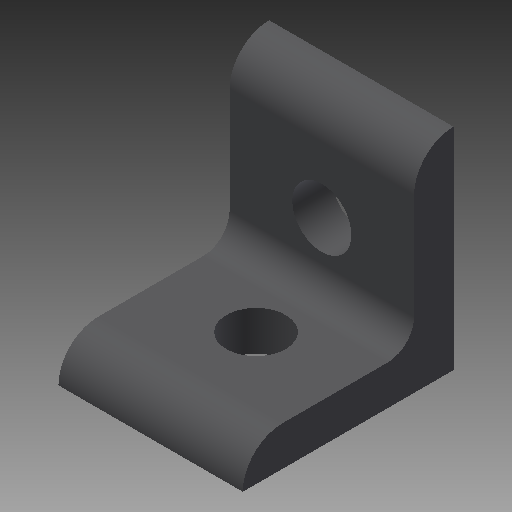
# Autodesk Inventor part: 4119
Saved by Autodesk Inventor 2017 SP1 (Build 210196100, 196)
## iProperties
Category: PARTsolutions
Company: 8020
Created: 2016-04-09
Part Number: 4119
Catalog Web Link: www.cadenas.de
Description: 4119, 4302-Joining Plates - 2 Hole Inside Corner Bracket
Vendor: 8020
Document SubType Name: Modeling
Designer: psAdmin
Manufacturer: 8020
Mass: 4.32354 g
Surface Area: 26.1381 cm^2
Volume: 4.32354 cm^3
Density: 1 g/cm^3
Material: Generic
Appearance: PSOLRGB-175-175-175
PSOL_IDENT_0: {$CADENAS_DATA\23d-libs\8020\inch\joining_plates\4119.prj},154 {VTYP=3D},{NB=4119},{LINA=4119},{NN=4
PSOL_IDENT_1: 119, 4302},{DATE=26.07.2013 08:18:18},{GEOMDATE=02.12.2011 13:06:00},{VERSION=},{LINEID=10},{LINESUB
PSOL_IDENT_2: ID=-1},{WBVAR=}  {NB=4119},{LINA=4119},{KT=DUMMY},{PN=4119},{A=0.875},{B=1.000},{C=1.000},{D=0.188},
PSOL_IDENT_3: {D1=0.18750},{E=0.281},{W=.025},{R=0.125}
NN: 4119, 4302
NT: Joining Plates - 2 Hole Inside Corner Bracket
NB: 4119
NBSYN: $PN.
LINA: 4119
PN: 4119
A: 0.875
B: 1.000
C: 1.000
D: 0.188
W: .025
SUPPLIER: 8020
ARTICLENO: 4119
BOMINFO: 4119
CREATOR: CADENAS GmbH
Title: 4119
Author: Cadenas PARTsolutions
Comments: Joining Plates - 2 Hole Inside Corner Bracket
Autodesk Inventor part; units mm, degrees
ref_plane "YZ Plane" through (0, 0, 0) normal (1, 0, 0) x (0, 1, 0)
ref_plane "XZ Plane" through (0, 0, 0) normal (0, 1, 0) x (-1, 0, 0)
ref_plane "XY Plane" through (0, 0, 0) normal (0, 0, 1) x (1, 0, 0)
sketch "Sketch_1" plane through (0, 0, 0) normal (1, 0, 0) x (0, 1, 0)
  line L0 (0, 25.4) -> (0, 0)
  line L1 (0, 0) -> (25.4, 0)
  arc A0 (25.4, 0) -> (20.6375, 4.7625) centre (20.6375, 0) ccw
  line L2 (20.6375, 4.7625) -> (7.9375, 4.7625)
  arc A1 (4.7625, 7.9375) -> (7.9375, 4.7625) centre (7.9375, 7.9375) ccw
  line L3 (4.7625, 7.9375) -> (4.7625, 20.6375)
  arc A2 (4.7625, 20.6375) -> (0, 25.4) centre (0, 20.6375) ccw
  constraints: 8 end point, 6 point on circle, 3 centre point
extrude "Extrusion1" add sketch "Sketch_1" along normal mid plane 22.225
sketch "Sketch2" plane through (11.1125, 0, 0) normal (0, 0, -1) x (-1, 0, 0)
  point P0 (11.1125, 12.7)
hole "Hole1" at (0, 12.7, 0) direction (0, 0, 1) diameter 7.1374 depth 4.7625
sketch "Sketch3" plane through (-11.1125, 0, 25.4) normal (0, -1, 0) x (1, 0, 0)
  point P0 (11.1125, -12.7)
hole "Hole2" at (0, 0, 12.7) direction (0, 1, 0) diameter 7.1374 depth 4.7625
body "Solid1"
